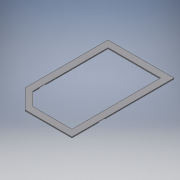
# Autodesk Inventor part: Backplate_V2
Saved by Autodesk Inventor 2016 SP2 (Build 200236200, 236)
## iProperties
Created: 2018-06-11
Part Number: Backplate_V2
Material: Generisch
Document SubType Name: Modeling
Designer: Nils
Density: 1 g/cm^3
Appearance: Vorgabe
Author: Nils
Autodesk Inventor part; units mm, degrees
ref_plane "YZ Plane" through (0, 0, 0) normal (1, 0, 0) x (0, 1, 0)
ref_plane "XZ Plane" through (0, 0, 0) normal (0, 1, 0) x (-1, 0, 0)
ref_plane "XY Plane" through (0, 0, 0) normal (0, 0, 1) x (1, 0, 0)
sketch "Skizze1" plane through (0, 0, 0) normal (0, 0, 1) x (1, 0, 0)
  line L0 (49.5001, 297.0913) -> (-49.5001, 297.0913) projected
  line L1 (49.5001, 143.8903) -> (49.5001, 297.0913) projected
  line L2 (-49.5001, 297.0913) -> (-49.5001, 143.8903) construction
  line L3 (-49.5001, 143.8903) -> (49.5001, 143.8903) construction
  circle A0 centre (-29.7001, 148.7389) radius 1.75 construction
  circle A1 centre (-44.8001, 148.7389) radius 1.75 construction
  circle A2 centre (-24.6237, 162.7718) radius 1.75 construction
  circle A3 centre (-20.9666, 159.2418) radius 1.75 construction
  circle A4 centre (44.5001, 148.8903) radius 2.5 construction
  circle A5 centre (44.5001, 220.1498) radius 2.5 construction
  circle A6 centre (-44.5001, 220.1498) radius 2.5 construction
  circle A7 centre (-44.5001, 292.0913) radius 2.5 construction
  circle A8 centre (44.5001, 292.0913) radius 2.5 construction
  line L4 (49.5001, 143.8903) -> (-20.6089, 143.8903)
  line L5 (-20.6089, 143.8903) -> (-49.5001, 172.7815)
  line L6 (-49.5001, 172.7815) -> (-49.5001, 297.0913)
  line L7 (-39.5001, 287.0913) -> (39.5001, 287.0913)
  line L8 (39.5001, 287.0913) -> (39.5001, 153.8903)
  line L9 (39.5001, 153.8903) -> (-19.2952, 153.8903)
  line L10 (-19.2952, 153.8903) -> (-39.5001, 174.0952)
  line L11 (-39.5001, 174.0952) -> (-39.5001, 287.0913)
  point P0 (0, 0)
  dimension "d0" = 135
  dimension "d1" = 8
  dimension "d2" = 3
  dimension "d3" = 10
  dimension "d4" = 10
  dimension "d5" = 10
  dimension "d6" = 10
  constraints: 16 end point, 3 perpendicular, 2 point on line, 1 collinear, 1 horizontal, 1 parallel
  measures "d0" angle of L5 L3
  measures "d1" distance between parallel lines of L5 L10
  measures "d2" distance from line of A0.centre L5
  measures "d3" distance between parallel lines of L3 L9
  measures "d4" distance between parallel lines of L1 L8
  measures "d5" distance between parallel lines of L2 L11
  measures "d6" distance between parallel lines of L0 L7
extrude "Extrusion1" add sketch "Skizze1" along normal blind 1.5
sketch "Skizze2" plane through (0, 0, 0) normal (0, 0, -1) x (-1, 0, 0)
  circle A0 centre (44.5001, 220.1498) radius 2.4 projected
  circle A1 centre (44.5001, 292.0913) radius 2.4 projected
  circle A2 centre (-44.5001, 292.0913) radius 2.4 projected
  circle A3 centre (-44.5001, 220.1498) radius 2.4 projected
  circle A4 centre (-44.5001, 148.8903) radius 2.4 projected
  circle A5 centre (40.1569, 169.0952) radius 2.5 construction
  circle A6 centre (40.1569, 169.0952) radius 2.4
  point P0 (0, 0)
  dimension "d19" = 4.8
  dimension "d20" = 4.8
  constraints: 1 centre point, 1 coincident
  measures "d19" diameter of A0
  measures "d20" diameter of A6
extrude "Extrusion2" add sketch "Skizze2" along normal blind 2.6
sketch "Skizze3" plane through (0, 0, 0) normal (0, 0, -1) x (-1, 0, 0)
  line L0 (-49.5001, 143.8903) -> (-49.5001, 297.0913) projected
  line L1 (-39.5001, 287.0913) -> (-39.5001, 153.8903) projected
  line L2 (-49.5001, 183.8903) -> (-39.5001, 183.8903)
  line L3 (-39.5001, 183.8903) -> (-39.5001, 193.8903)
  line L4 (-39.5001, 193.8903) -> (-49.5001, 193.8903)
  line L5 (-49.5001, 193.8903) -> (-49.5001, 183.8903)
  line L6 (39.5001, 287.0913) -> (39.5001, 174.0952) projected
  line L7 (49.5001, 297.0913) -> (49.5001, 172.7815) projected
  line L8 (39.5001, 183.8903) -> (49.5001, 183.8903)
  line L9 (49.5001, 183.8903) -> (49.5001, 193.8903)
  line L10 (49.5001, 193.8903) -> (39.5001, 193.8903)
  line L11 (39.5001, 193.8903) -> (39.5001, 183.8903)
  line L12 (39.5001, 174.0952) -> (19.2952, 153.8903) projected
  line L13 (20.7094, 155.3045) -> (26.3662, 149.6477)
  line L14 (49.5001, 172.7815) -> (20.6089, 143.8903) projected
  line L15 (26.3662, 149.6477) -> (33.4373, 156.7188)
  line L16 (33.4373, 156.7188) -> (27.7805, 162.3756)
  line L17 (27.7805, 162.3756) -> (20.7094, 155.3045)
  line L18 (20.6089, 143.8903) -> (-49.5001, 143.8903) projected
  point P0 (0, 0)
  dimension "d11" = 10
  dimension "d12" = 10
  dimension "d13" = 10
  dimension "d14" = 0
  dimension "d15" = 40
  dimension "d16" = 2
  constraints: 24 end point, 8 point on line, 4 parallel, 3 perpendicular, 2 horizontal, 1 collinear
  measures "d11" distance between parallel lines of L2 L4
  measures "d12" distance between parallel lines of L16 L13
  measures "d13" distance between parallel lines of L10 L8
  measures "d14" distance between parallel lines of L8 L2
  measures "d15" distance between parallel lines of L18 L2
  measures "d16" distance from line of L12.end L13
extrude "Extrusion3" cut sketch "Skizze3" against normal blind 1 contours L0 L4 L1 L2 | L13 L12 L16 L14 | L8 L6 L10 L7
equation "\"d4\" = d3"
equation "\"d5\" = d3"
equation "\"d6\" = d3"
equation "\"d20\" = d19"
equation "\"d12\" = d11"
equation "\"d13\" = d11"
